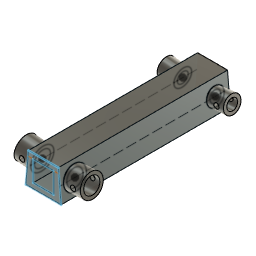
Wing to mainrod connector v4 (Autodesk Fusion 360 design; units mm, degrees)
Autodesk Fusion 360 part; units mm, degrees
sketch "Main cross-section sketch" plane through (0, 0, 0) normal (0, 1, 0) x (1, 0, 0)
  line L0 (3.8558, -6.289) -> (-8.3442, -6.289)
  line L1 (-8.3442, -6.289) -> (-8.3442, 5.911)
  line L2 (-8.3442, 5.911) -> (3.8558, 5.911)
  line L3 (3.8558, 5.911) -> (3.8558, -6.289)
  line L4 (6.5933, -9.289) -> (-11.0818, -9.289)
  line L5 (-11.0818, -9.289) -> (-12.6741, 8.911)
  line L6 (-12.6741, 8.911) -> (8.1856, 8.911)
  line L7 (8.1856, 8.911) -> (6.5933, -9.289)
  line L8 (-11.0818, -9.289) -> (6.5933, -9.289)
  line L9 (-8.3442, -6.289) -> (-11.3442, -6.289) construction
  line L10 (3.8558, -6.289) -> (6.8558, -6.289) construction
  dimension "d13" = 85
  dimension "d14" = 85
  dimension "d20" = 3
  dimension "d22" = 3
  dimension "d25" = 3
  dimension "d26" = 12.2
  constraint equal L1 L2
  constraint horizontal L8
  constraint horizontal L0
  constraint equal L0 L1
  constraint coincident L5 L9.end
  constraint vertical L1
  constraint horizontal L9
  constraint vertical L3
  constraint equal L0 L3
  constraint coincident L7 L10.end
  constraint parallel L0 L10
  constraint equal L9 L10
  measures "d13" angle of L5 L6
  measures "d14" angle of L6 L7
  measures "d20" distance of L0.end L9.end
  measures "d22" distance of L0 L4
  measures "d25" distance of L2 L6
  measures "d26" distance of L0.start L2.end
extrude "Extrude1" add sketch "Main cross-section sketch" along normal blind 100
sketch "Right side sketch" plane through (7.3497, 0, 0.643) normal (0.996195, 0, 0.087156) x (0, 1, 0)
  line L0 (0, 8.679) -> (0, -9.5905)
  line L1 (0, -9.5905) -> (100, -9.5905)
  line L2 (100, -9.5905) -> (100, 8.679)
  line L3 (100, 8.679) -> (0, 8.679)
  circle A0 centre (9, -0.4557) radius 4.775
  circle A1 centre (92.0226, -0.4557) radius 3.19
  line L4 (9, -0.4557) -> (0, -0.4557) construction
  line L5 (9, -0.4557) -> (92.0226, -0.4557) construction
  line L6 (92.0226, -0.4557) -> (100, -0.4557) construction
  circle A2 centre (9, -0.4557) radius 6.775
  circle A3 centre (92.0226, -0.4557) radius 5.19
  dimension "d29" = 83.0226
  dimension "d31" = 9.55
  dimension "d32" = 6.38
  dimension "d35" = 13.55
  dimension "d36" = 10.38
  dimension "d44" = 9
  constraint midpoint L0 L4.end
  constraint coincident A0.centre L4.start
  constraint coincident A1.centre L5.end
  constraint parallel L4 L5
  constraint midpoint L2 L6.end
  constraint perpendicular L2 L6
  constraint parallel L5 L6
  constraint concentric A0 A2
  constraint concentric A1 A3
  measures "d29" distance of A0.centre A1.centre
  measures "d31" diameter of A0
  measures "d32" diameter of A1
  measures "d35" diameter of A2
  measures "d36" diameter of A3
  measures "d44" distance of L0 A0.centre
extrude "Extrude2" add sketch "Right side sketch" along normal blind 10 contours A2 | A3
sketch "Left side sketch" plane through (-11.8041, 0, 1.0327) normal (-0.996195, 0, 0.087156) x (0, -1, 0)
  line L0 (0, -9.9817) -> (0, 8.2879)
  line L1 (0, 8.2879) -> (-100, 8.2879)
  line L2 (-100, 8.2879) -> (-100, -9.9817)
  line L3 (-100, -9.9817) -> (0, -9.9817)
  circle A0 centre (-92.0226, -0.8469) radius 5.19
  circle A1 centre (-92.0226, -0.8469) radius 3.19
  circle A2 centre (-9, -0.8469) radius 4.775
  circle A3 centre (-9, -0.8469) radius 6.775
  line L4 (-100, -0.8469) -> (0, -0.8469) construction
  dimension "d40" = 9.55
  dimension "d41" = 6.38
  dimension "d42" = 13.55
  dimension "d43" = 10.38
  dimension "d46" = 83.0226
  dimension "d47" = 9
  constraint concentric A2 A3
  constraint concentric A0 A1
  constraint midpoint L2 L4.start
  constraint midpoint L0 L4.end
  constraint coincident A2.centre L4
  constraint coincident A0.centre L4
  measures "d40" diameter of A2
  measures "d41" diameter of A1
  measures "d42" diameter of A3
  measures "d43" diameter of A0
  measures "d46" distance of A2.centre A0.centre
  measures "d47" distance of L0 A2.centre
extrude "Extrude3" add sketch "Left side sketch" along normal blind 10 contours A0 | A3
hole "Hole1" at (-16.9554, 86.8326, 0.6333) direction (0, 1, 0) diameter 3.1 depth 12 tip angle 180
hole "Hole2" at (13.1771, 86.8326, 0.6954) direction (0, 1, 0) diameter 3.1 depth 12 tip angle 180
hole "Hole3" at (-17.1859, 2.225, 0.6534) direction (0, 1, 0) diameter 3.1 depth 18 tip angle 180
hole "Hole4" at (13.0025, 2.225, 0.6801) direction (0, 1, 0) diameter 3.1 depth 18 tip angle 180
equation "d35 = 9.55 mm + 4 mm"
equation "d36 = 6.38 mm + 4 mm"
equation "d42 = 9.55 mm + 4 mm"
equation "d43 = 6.38 mm + 4 mm"
